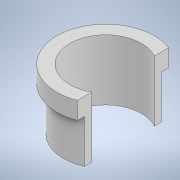
# Autodesk Inventor part: adapter
Saved by Autodesk Inventor 2022 (Build 260153000, 153)
## iProperties
Created: 2021-12-30
Part Number: adapter
Material: Genérico
Document SubType Name: Modeling
Designer: JK
Density: 1 g/cm^3
Appearance: Valor por defecto
Author: JK
Autodesk Inventor part; units mm, degrees
ref_plane "YZ Plane" through (0, 0, 0) normal (1, 0, 0) x (0, 1, 0)
ref_plane "XZ Plane" through (0, 0, 0) normal (0, 1, 0) x (-1, 0, 0)
ref_plane "XY Plane" through (0, 0, 0) normal (0, 0, 1) x (1, 0, 0)
sketch "Boceto1" plane through (0, 0, 0) normal (0, 1, 0) x (-1, 0, 0)
  circle A0 centre (0, 0) radius 1.65
  circle A1 centre (0, 0) radius 1.95
  line L0 (-0.8, 1.7783) -> (-0.8, -1.7783)
  point P0 (-0.8, 1.4431)
  point P1 (-0.8, -1.4431)
  dimension "d0" = 3.3
  dimension "d1" = 0.3
  dimension "d2" = 0.8
  constraints: 2 centre point, 2 coincident, 2 end point, 2 point on circle, 1 vertical
  measures "d0" diameter of A0
  measures "d1" radial gap between concentric circles of A1 A0
  measures "d2" distance from line of point (0, 0) L0
extrude "Extrusión1" add sketch "Boceto1" along normal blind 2 contours A0 L0 A1 picked at (1.8153, 0.2861)
sketch "Boceto2" plane through (0, 2, 0) normal (0, 1, 0) x (1, 0, 0)
  arc A0 (0.8, 1.4431) -> (0.8, -1.4431) centre (0, 0) ccw projected
  circle A1 centre (0, 0) radius 2.25
  line L0 (0.8, -2.103) -> (0.8, 2.103)
  line L1 (0.8, 1.4431) -> (0.8, 1.7783) projected
  point P0 (0.8, 1.4431)
  point P1 (0.8, -1.4431)
  dimension "d5" = 0.6
  constraints: 2 end point, 2 point on circle, 1 centre point, 1 coincident, 1 collinear, 1 vertical
  measures "d5" radial gap between concentric circles of A1 A0
extrude "Extrusión2" add sketch "Boceto2" along normal blind 0.8 contours A0 L0 A1
